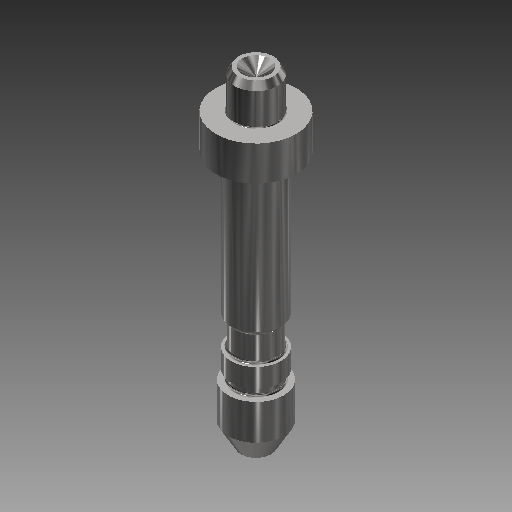
# Autodesk Inventor part: 100-03
Saved by Autodesk Inventor 2019 (Build 230136000, 136)
## iProperties
Company: Autodesk Inc.
Created: 2007-11-14
Part Number: 100-03
Document SubType Name: Modeling
Designer: Autodesk Inc.
Density: 8 g/cm^3
Mass: 33.5583 g
Surface Area: 20.919 cm^2
Volume: 4.19479 cm^3
Material: Stainless Steel
Description: SIDE HANDLE PIVOT PIN
Appearance: Steel - Polished
Component Category: Side Component
Author: Inventor
Autodesk Inventor part; units mm, degrees
ref_plane "YZ Plane" through (0, 0, 0) normal (1, 0, 0) x (0, 1, 0)
ref_plane "XZ Plane" through (0, 0, 0) normal (0, 1, 0) x (-1, 0, 0)
ref_plane "XY Plane" through (0, 0, 0) normal (0, 0, 1) x (1, 0, 0)
sketch "Sketch1" plane through (0, 0, 0) normal (0, 0, 1) x (1, 0, 0)
  line L0 (0, 18.9) -> (0, -64.4) projected
  line L1 (-1.45, 0) -> (8.7, 0) projected
  line L2 (0, 5.2495) -> (2.5, 7)
  line L3 (2.5, 7) -> (3.157, 7)
  line L4 (3.157, 7) -> (3.85, 5.8)
  line L5 (3.85, 5.8) -> (3.85, 0)
  line L6 (3.85, 0) -> (7.25, 0)
  line L7 (7.25, 0) -> (7.25, -6.3)
  line L8 (7.25, -6.3) -> (4.5, -6.3)
  line L9 (4.5, -6.3) -> (4.5, -31.575)
  line L10 (4.5, -31.575) -> (3.75, -32.325)
  line L11 (3.75, -32.325) -> (3.75, -37)
  line L12 (3.75, -37) -> (4.5, -37)
  line L13 (4.5, -37) -> (4.5, -40.4)
  line L14 (4.5, -40.4) -> (3.75, -40.4)
  line L15 (3.75, -40.4) -> (3.75, -42.1)
  line L16 (3.75, -42.1) -> (5.025, -42.1)
  line L17 (5.025, -42.1) -> (5.025, -48.5)
  line L18 (5.025, -48.5) -> (2.7156, -52.5)
  line L19 (2.7156, -52.5) -> (1.7713, -52.5)
  line L20 (1.7713, -52.5) -> (0, -51.2597)
  line L21 (0, -51.2597) -> (0, 5.2495)
  point P0 (0, 0)
  dimension "d0" = 7
  dimension "d1" = 3.85
  dimension "d2" = 1.2
  dimension "d3" = 3.157
  dimension "d4" = 35
  dimension "d5" = 2.5
  dimension "d7" = 7.25
  dimension "d8" = 6.3
  dimension "d9" = 4.5
  dimension "d10" = 3.75
  dimension "d13" = 45
  dimension "d14" = 5.425
  dimension "d15" = 4.5
  dimension "d16" = 3.4
  dimension "d17" = 3.75
  dimension "d18" = 1.7
  dimension "d19" = 5.025
  dimension "d20" = 52.5
  dimension "d21" = 35
  dimension "d22" = 30
  dimension "d23" = 6.4
  dimension "d28" = 0.9443
  dimension "d29" = 4
  constraints: 40 end point, 8 perpendicular, 5 parallel, 4 point on line, 1 collinear
  measures "d0" distance between parallel lines of L3 L1
  measures "d1" distance between parallel lines of L21 L5
  measures "d2" vertical distance of L3.end L4.end
  measures "d3" distance from line of L0 L3.end
  measures "d4" angle of L3 L2
  measures "d5" distance from line of L0 L2.end
  measures "d7" distance between parallel lines of L7 L0
  measures "d8" distance of L6.end L7.end
  measures "d9" distance between parallel lines of L21 L9
  measures "d10" distance between parallel lines of L21 L11
  measures "d13" angle of L10 L9
  measures "d14" distance from line of L9.end L12
  measures "d15" distance between parallel lines of L21 L13
  measures "d16" distance of L12.end L13.end
  measures "d17" distance between parallel lines of L21 L15
  measures "d18" distance of L14.end L15.end
  measures "d19" distance between parallel lines of L21 L17
  measures "d20" distance between parallel lines of L6 L19
  measures "d21" angle of L19 L20
  measures "d22" angle of L17 L18
  measures "d23" distance of L16.end L17.end
  measures "d28" distance of L18.end L19.end
  measures "d29" vertical distance of L18.end L17.end
revolve "Revolution1" add sketch "Sketch1" angle 360 about axis through (0, -51.2597, 0) along (0, 1, 0)
fillet "Fillet1" radius 0.5 5 edges at (-3.75, -42.1, 0) (-3.75, -40.4, 0) (-3.75, -32.325, 0) (-4.5, -6.3, 0) (-3.75, -37, 0)
fillet "Fillet2" radius 0.25 1 edges at (-3.85, 0, 0)
body "Solid1"
